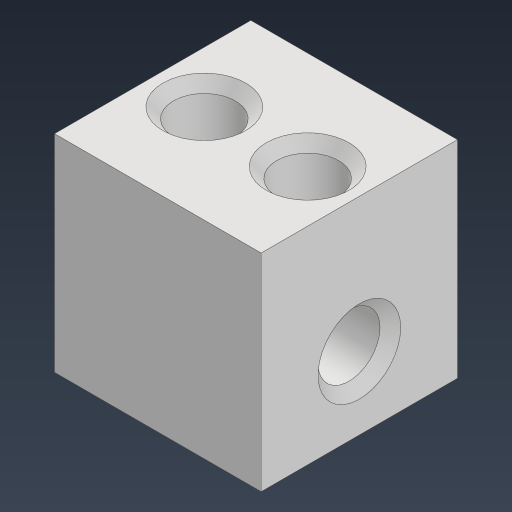
# Autodesk Inventor part: glue_test_PULLING_2
Saved by Autodesk Inventor 2023 (Build 270158000, 158)
## iProperties
Created: 2025-12-21
Part Number: glue_test_PULLING_2
Material: Generic
Document SubType Name: Modeling
Designer: szymo
Density: 1 g/cm^3
Appearance: Default
Author: szymo
Autodesk Inventor part; units mm, degrees
ref_plane "YZ Plane" through (0, 0, 0) normal (1, 0, 0) x (0, 1, 0)
ref_plane "XZ Plane" through (0, 0, 0) normal (0, 1, 0) x (-1, 0, 0)
ref_plane "XY Plane" through (0, 0, 0) normal (0, 0, 1) x (1, 0, 0)
sketch "Sketch1" plane through (0, 0, 0) normal (0, 1, 0) x (-1, 0, 0)
  line L0 (-5, 4.75) -> (5, 4.75)
  line L1 (5, 4.75) -> (5, -4.75)
  line L2 (5, -4.75) -> (-5, -4.75)
  line L3 (-5, -4.75) -> (-5, 4.75)
  line L4 (-5, 4.75) -> (5, -4.75) construction
  line L5 (5, 4.75) -> (-5, -4.75) construction
  line L6 (-5, 0) -> (5, 0) construction
  circle A0 centre (-2.5, 0) radius 1.5
  circle A1 centre (2.5, 0) radius 1.5
  point P0 (0, 0)
  point P1 (0, 0)
  dimension "d0" = 10
  dimension "d1" = 9.5
  dimension "d2" = 3
  dimension "d3" = 3
  dimension "d4" = 2.5
  dimension "d5" = 2.5
  dimension "d6" = 2.5
  dimension "d7" = 2.5
  constraints: 14 end point, 5 midpoint, 2 centre point, 2 parallel, 2 point on line, 1 horizontal, 1 perpendicular
  measures "d0" distance of L1.end L2.end
  measures "d1" distance of L0.end L1.end
  measures "d2" diameter of A0
  measures "d3" diameter of A1
  measures "d4" distance from line of L3 A0.centre
  measures "d5" distance of point (0, 0) A0.centre
  measures "d6" distance of point (0, 0) A1.centre
  measures "d7" distance of A1.centre L6.end
extrude "Extrusion1" add sketch "Sketch1" along normal blind 10
extrude "Extrusion2" add sketch "Sketch1" along normal blind 6 contours A0 | A1
sketch "Sketch2" plane through (5, 0, 4.75) normal (1, 0, 0) x (0, 0, -1)
  line L0 (0, 0) -> (9.5, 0) projected
  line L1 (9.5, 0) -> (9.5, 10) projected
  line L2 (0, 10) -> (9.5, 10) projected
  line L3 (0, 0) -> (0, 10) projected
  circle A0 centre (4.75, 3.5) radius 1.5
  point P0 (4.75, 0)
  dimension "d12" = 3
  dimension "d13" = 3.5
  dimension "d14" = 4.75
  dimension "d15" = 4.75
  constraints: 1 centre point
  measures "d12" diameter of A0
  measures "d13" distance from line of L0 A0.centre
  measures "d14" distance from line of L3 A0.centre
  measures "d15" distance from line of L1 A0.centre
extrude "Extrusion3" cut sketch "Sketch2" against normal through all contours A0
chamfer "Chamfer1" distance 0.5 angle 45 4 edges at (4, 10, 0) (-1, 10, 0) (-5, 3.5, 1.5) (5, 3.5, 1.5)
equation "\"d4\" = d5"
equation "\"d6\" = d7"
equation "\"d14\" = d15"
body "Solid1"
